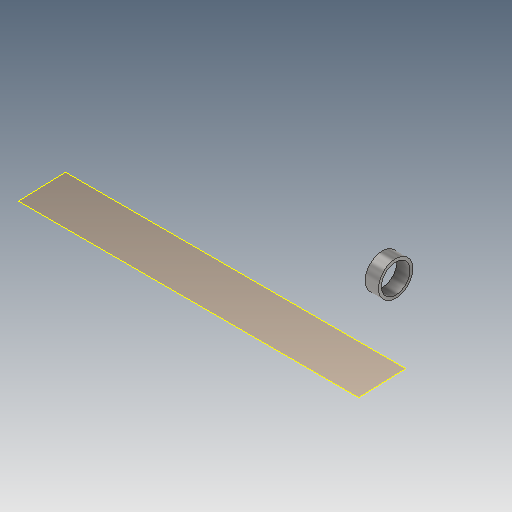
# Autodesk Inventor part: 高速轴套筒1
Saved by Autodesk Inventor 2025 (Build 290162000, 162)
## iProperties
Created: 2025-03-20
Part Number: 高速轴套筒1
Material: 钢，软
Document SubType Name: Modeling
Designer: liukan
Density: 7.85 g/cm^3
Appearance: 半抛光
Author: liukan
Autodesk Inventor part; units mm, degrees
ref_plane "YZ Plane" through (0, 0, 0) normal (1, 0, 0) x (0, 1, 0)
ref_plane "XZ Plane" through (0, 0, 0) normal (0, 1, 0) x (-1, 0, 0)
ref_plane "XY Plane" through (0, 0, 0) normal (0, 0, 1) x (1, 0, 0)
ref_plane "工作平面1" through (-9.0747, 111.0101, -65.7955) normal (0, 0.9995, 0.0326) x (-1, 0, 0)
sketch "草图1" plane through (-9.0747, 111.0101, -65.7955) normal (0, 0.9995, 0.0326) x (-1, 0, 0)
  line L0 (-242.343, -78.4652) -> (-242.343, -119.6652) projected
  line L1 (-256.343, -114.0652) -> (-256.343, -84.0652) projected
  line L2 (-258.343, -119.0652) -> (-258.343, -79.0652) projected
  line L3 (-256.343, 15) -> (-95.5, 15) construction
  line L4 (-256.343, -15) -> (-95.5, -15)
  line L5 (-242.343, -81.0652) -> (-256.343, -81.0652)
  line L6 (-256.343, -81.0652) -> (-256.343, -84.0652)
  line L7 (-256.343, -84.0652) -> (-242.343, -84.0652)
  line L8 (-242.343, -84.0652) -> (-242.343, -81.0652)
  line L9 (-242.343, -99.0652) -> (-256.343, -99.0652) construction
  line L10 (-242.343, -99.0652) -> (-256.343, -99.0652)
  point P0 (-9.0747, 69.3815)
  point P1 (-95.5, -15)
  point P2 (-249.343, -99.0652)
  point P3 (-242.343, -84.0652)
  dimension "d0" = 18
  constraints: 16 end point, 3 equal length, 3 horizontal, 3 midpoint, 1 perpendicular, 1 point on line, 2 other
  measures "d0" distance from line of point (-249.343, -99.065) L5
revolve "旋转1" add sketch "草图1" angle 360 about axis through (233.2683, 114.2415, -164.808) along (1, 0, 0) contours L0 L7 L6 L5
